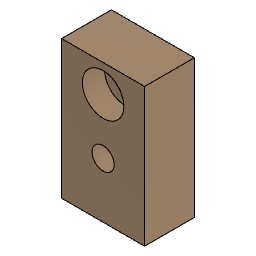
Standoff BR (Autodesk Fusion 360 design; units mm, degrees)
Autodesk Fusion 360 part; units mm, degrees
sketch "Front" plane through (0, 0, 0) normal (0, 1, 0) x (1, 0, 0)
  line L0 (-15, -25) -> (15, -25)
  line L1 (15, -25) -> (15, 25)
  line L2 (15, 25) -> (-15, 25)
  line L3 (-15, 25) -> (-15, -25)
  line L4 (0, -25) -> (0, 25) construction
  circle A0 centre (0, -15) radius 4
  circle A1 centre (0, 5) radius 4
  circle A2 centre (0, -15) radius 7.5
  dimension "d13" = 30
  dimension "d14" = 50
  dimension "d17" = 8
  dimension "d18" = 8
  dimension "d22" = 20
  dimension "d23" = 10
  dimension "d25" = 15
  constraint horizontal L0
  constraint vertical L1
  constraint horizontal L2
  constraint vertical L3
  constraint midpoint L0 L4.start
  constraint midpoint L2 L4.end
  constraint coincident L4 A0.centre
  constraint coincident L4 A1.centre
  constraint concentric A0 A2
  measures "d13" distance of L0.start L0.end
  measures "d14" distance of L0.start L2.end
  measures "d17" diameter of A0
  measures "d18" diameter of A1
  measures "d22" distance of A0.centre A1.centre
  measures "d23" distance of L0 A0.centre
  measures "d25" diameter of A2
extrude "Extrude3" add sketch "Front" against normal blind 10 contours A2
extrude "Extrude4" add sketch "Front" against normal blind 18 contours L0 L1 L2 L3
named bodies: "Standoff BR"
